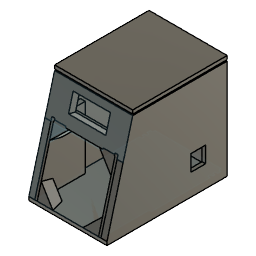
3rd_Seisaku_Alarm (Autodesk Fusion 360 design; units mm, degrees)
Autodesk Fusion 360 part; units mm, degrees
sketch "スケッチ1" plane through (0, 0, 0) normal (0, 0, 1) x (1, 0, 0)
  line L0 (0, 0) -> (3, 0)
  line L1 (3, 0) -> (3, 100)
  line L2 (3, 100) -> (0, 100)
  line L3 (0, 100) -> (0, 0)
  line L4 (3, 100) -> (62, 100)
  line L5 (62, 100) -> (62, 97)
  line L6 (62, 97) -> (3, 97)
  line L7 (3, 97) -> (3, 100)
  line L8 (65.000001, 100.000001) -> (62.000001, 100.000001)
  line L9 (62.000001, 100.000001) -> (62.000001, 0.000001)
  line L10 (62.000001, 0.000001) -> (65.000001, 0.000001)
  line L11 (65.000001, 0.000001) -> (65.000001, 100.000001)
  dimension "d1" = 100
  dimension "d2" = 59
  dimension "d3" = 3
  dimension "d4" = 3
  dimension "d5" = 100
  constraint horizontal L0
  constraint vertical L1
  constraint horizontal L2
  constraint vertical L3
  constraint coincident L0.start L3.end
  constraint horizontal L4
  constraint vertical L5
  constraint horizontal L6
  constraint vertical L7
  constraint horizontal L8
  constraint vertical L9
  constraint horizontal L10
  constraint vertical L11
  measures "d1" distance of L0.start L2.end
  measures "d2" distance of L1.end L4.end
  measures "d3" distance of L1.end L6.end
extrude "押し出し1" add sketch "スケッチ1" along normal blind 80 makes body 1
sketch "スケッチ2" plane through (65.000001, 0, 0) normal (1, 0, 0) x (0, 1, 0)
  line L0 (0.000001, 0) -> (100.000001, 0)
  line L1 (100.000001, 0) -> (100.000001, 80)
  line L2 (100.000001, 80) -> (0.000001, 80)
  line L3 (0.000001, 80) -> (0.000001, 0)
  line L4 (0.000001, 0) -> (22.116636, 82.540402)
  line L5 (0.000001, 0) -> (85.452114, 0) construction
  line L6 (22.116636, 82.540402) -> (0, 82.540402)
  line L7 (0, 82.540402) -> (0.000001, 0)
  dimension "d8" = 75
  constraint horizontal L5
  constraint perpendicular L3 L6
  measures "d8" angle of L4 L5
extrude "押し出し2" cut sketch "スケッチ2" against normal blind 115 contours L2 L3 L4 L7 picked at (7.145313, 53.333333) bodies 1
sketch "スケッチ3" plane through (0, 0, 0) normal (0, 0, 1) x (1, 0, 0)
  line L0 (65, 100) -> (0, 100)
  line L1 (0, 100) -> (0, 0)
  line L2 (0, 0) -> (65, 0)
  line L3 (65, 0) -> (65, 100)
  constraint horizontal L0
  constraint vertical L1
  constraint horizontal L2
  constraint vertical L3
  constraint coincident L1.end L2.start
extrude "押し出し3" add sketch "スケッチ3" against normal blind 3 bodies 1
sketch "スケッチ4" plane through (0, 0, 0) normal (0, 1, 0) x (1, 0, 0)
  line L0 (0, 0) -> (5, 0)
  line L1 (5, 0) -> (5, -50)
  line L2 (5, -50) -> (0, -50)
  line L3 (0, -50) -> (0, 0)
  line L4 (65.000001, 0) -> (60.000001, 0)
  line L5 (60.000001, 0) -> (60.000001, -50)
  line L6 (60.000001, -50) -> (65.000001, -50)
  line L7 (65.000001, -50) -> (65.000001, 0)
  dimension "d13" = 5
  dimension "d14" = 50
  dimension "d15" = 5
  dimension "d16" = 50
  constraint horizontal L0
  constraint vertical L1
  constraint horizontal L2
  constraint vertical L3
  constraint coincident L0.start L3.end
  constraint horizontal L4
  constraint vertical L5
  constraint horizontal L6
  constraint vertical L7
  measures "d13" distance of L0.start L0.end
  measures "d14" distance of L0.start L2.end
extrude "押し出し4" add sketch "スケッチ4" along normal blind 40 bodies 1
sketch "スケッチ5" plane through (65.000001, 0, 0) normal (1, 0, 0) x (0, 1, 0)
  line L0 (0, 50) -> (0, -3)
  line L1 (0, -3) -> (100, -3)
  line L2 (100, -3) -> (100.000001, 80)
  line L3 (100.000001, 80) -> (21.435937, 80)
  line L4 (21.435937, 80) -> (13.397461, 50)
  line L5 (13.397461, 50) -> (0, 50)
  line L6 (0, 0) -> (14.246435, 53.168413)
  line L7 (14.246435, 53.168413) -> (0, 53.168413)
  line L8 (0, 53.168413) -> (0, 0)
  constraint coincident L6.start L8.end
  constraint parallel L5 L7
  constraint perpendicular L7 L8
extrude "押し出し5" cut sketch "スケッチ5" against normal blind 77 contours L0 L5 L6 L8 picked at (4.46582, 33.333333) bodies 1
sketch "スケッチ6" plane through (0, 0, 0) normal (0, -0.965926, 0.258819) x (1, 0, 0)
  line L0 (5, 0) -> (5, 51.763809)
  line L1 (5, 51.763809) -> (3, 51.763809)
  line L2 (3, 51.763809) -> (0, 51.763809)
  line L3 (0, 51.763809) -> (0, 0)
  line L4 (0, 0) -> (5, 0)
  line L5 (5, 51.763809) -> (17, 51.763809)
  line L6 (5, 51.763809) -> (5, 39.763809)
  line L7 (17, 51.763809) -> (5, 39.763809)
  line L8 (59.943204, 51.763809) -> (47.943204, 51.763809)
  line L9 (59.943204, 51.763809) -> (59.943204, 39.763809)
  line L10 (59.943204, 39.763809) -> (47.943204, 51.763809)
  line L11 (5, 0) -> (5, 12)
  line L12 (5, 0) -> (17, 0)
  line L13 (5, 12) -> (17, 0)
  line L14 (60.000001, 0) -> (48.000001, 0)
  line L15 (60.000001, 0) -> (60.000001, 12)
  line L16 (60.000001, 12) -> (48.000001, 0)
  dimension "d21" = 12
  dimension "d22" = 12
  dimension "d23" = 12
  dimension "d24" = 12
  dimension "d25" = 12
  dimension "d26" = 12
  dimension "d27" = 12
  dimension "d28" = 12
  constraint perpendicular L0 L5
  constraint perpendicular L6 L8
  constraint perpendicular L8 L9
  constraint coincident L0.start L4.end
  constraint perpendicular L4 L11
  constraint perpendicular L11 L12
  constraint perpendicular L11 L14
  constraint perpendicular L14 L15
  measures "d25" distance of L0.start L11.end
  measures "d26" distance of L0.start L12.end
extrude "押し出し6" add sketch "スケッチ6" against normal blind 5 separate body contours L0 L11 L12 L13 | L0 L5 L6 L7 | L8 L9 L10 | L14 L15 L16 picked at (9, 4) picked at (9, 47.763809) picked at (55.943204, 47.763809) picked at (56.000001, 4) makes body 2 at (13, 2.645153, 3.432338) makes body 3 at (56.000001, 3.680429, 7.296042) makes body 4 at (9, 14.546661, 41.409863) makes body 5 at (55.943204, 12.936785, 41.841228)
sketch "スケッチ7" plane through (5, 0, 0) normal (1, 0, 0) x (0, 1, 0)
  line L0 (13.397461, 50) -> (0, 0)
  line L1 (0, 0) -> (40, 0)
  line L2 (40, 0) -> (40, 50)
  line L3 (40, 50) -> (13.397461, 50)
sketch "スケッチ8" plane through (5, 0, 0) normal (1, 0, 0) x (0, 1, 0)
extrude "押し出し7" add 2 faces at (9, 15.007337, 49.568635) (55.943204, 15.007337, 49.568635) along direction (0, 0.25881907, 0.96592582) blind 2 on bodies 4 5 bodies 1 2 3 5 4
sketch "スケッチ9" plane through (0, 0, 0) normal (0, -0.965926, 0.258819) x (1, 0, 0)
  line L0 (5, 51.763809) -> (3, 51.763809)
  line L1 (3, 51.763809) -> (0, 51.763809)
  line L2 (0, 51.763809) -> (0, 0)
  line L3 (0, 0) -> (5, 0)
  line L4 (5, 0) -> (5, 39.763809)
  line L5 (5, 39.763809) -> (17, 51.763809)
  line L6 (17, 51.763809) -> (17, 53.763809)
  line L7 (17, 53.763809) -> (5, 53.763809)
  line L8 (5, 53.763809) -> (5, 51.763809)
  line L9 (3, 51.763809) -> (62.000001, 51.763809)
  line L10 (62.000001, 51.763809) -> (62.000001, 55.000001)
  line L11 (62.000001, 55.000001) -> (3, 55.000001)
  line L12 (3, 55.000001) -> (3, 51.763809)
  constraint horizontal L9
  constraint vertical L10
  constraint horizontal L11
  constraint vertical L12
sketch "スケッチ10" plane through (3, 0, 0) normal (1, 0, 0) x (0, 1, 0)
  line L0 (13.397461, 50) -> (40, 50)
  line L1 (40, 50) -> (40, 0)
  line L2 (40, 0) -> (97, 0)
  line L3 (97, 0) -> (97, 80)
  line L4 (97, 80) -> (21.435937, 80)
  line L5 (21.435937, 80) -> (13.397461, 50)
  line L6 (40, 50) -> (13, 50)
  line L7 (13, 50) -> (13, 53.000001)
  line L8 (13, 53.000001) -> (40, 53.000001)
  line L9 (40, 53.000001) -> (40, 50)
  constraint horizontal L6
  constraint vertical L7
  constraint horizontal L8
  constraint vertical L9
  constraint coincident L0.end L1.start
extrude "押し出し8" add sketch "スケッチ10" along normal blind 59 contours L0 L5 L6 L8 L9 picked at (22.532923, 51) bodies 1 5
sketch "スケッチ11" plane through (0, 0, 53.000001) normal (0, 0, 1) x (-1, 0, 0)
  line L0 (-3, -40) -> (-3, -14.201309)
  line L1 (-3, -14.201309) -> (-62, -14.201309)
  line L2 (-62, -14.201309) -> (-62, -40)
  line L3 (-62, -40) -> (-3, -40)
  line L4 (-62, -40) -> (-3, -40)
  line L5 (-3, -40) -> (-3, -30)
  line L6 (-3, -30) -> (-62, -30)
  line L7 (-62, -30) -> (-62, -40)
  constraint horizontal L4
  constraint vertical L5
  constraint horizontal L6
  constraint vertical L7
  constraint coincident L0 L5.end
  constraint coincident L2.end L3.start
extrude "押し出し9" cut sketch "スケッチ11" against normal blind 3 contours L0 L2 L3 L4 L5 L6 L7 picked at (-42.333333, -36.666667) bodies 1
sketch "スケッチ12" plane through (0, 0, 50.000001) normal (0, 0, 1) x (-1, 0, 0)
  line L0 (-5, -30) -> (-5, -40)
  line L1 (-5, -40) -> (-3, -40)
  line L2 (-3, -40) -> (-3, -30)
  line L3 (-3, -30) -> (-5, -30)
  line L4 (-3, -30) -> (-5, -30)
  line L5 (-5, -30) -> (-5, -40)
  line L6 (-5, -40) -> (-3, -40)
  line L7 (-3, -40) -> (-3, -30)
  line L8 (-60.000001, -40.000001) -> (-62.000001, -40.000001)
  line L9 (-62.000001, -40.000001) -> (-62.000001, -30)
  line L10 (-62.000001, -30) -> (-60.000001, -30)
  line L11 (-60.000001, -30) -> (-60.000001, -40.000001)
  constraint horizontal L4
  constraint vertical L5
  constraint horizontal L6
  constraint vertical L7
  constraint coincident L0.end L1.start
  constraint coincident L2.end L3.start
  constraint horizontal L8
  constraint vertical L9
  constraint horizontal L10
  constraint vertical L11
extrude "押し出し10" add sketch "スケッチ12" along normal blind 3 bodies 1
extrude "押し出し11" cut 1 faces at (42.333333, 97, 26.666667) along direction (0, 1, 0) blind 49 on bodies 1 bodies 1
sketch "スケッチ13" plane through (0, 0.000001, 0) normal (0, -0.965926, 0.258819) x (1, 0, 0)
  line L0 (0, 51.763809) -> (5, 51.763809)
  line L1 (5, 51.763809) -> (5, 53.763809)
  line L2 (5, 53.763809) -> (17, 53.763809)
  line L3 (17, 53.763809) -> (17, 51.763809)
  line L4 (17, 51.763809) -> (47.943204, 51.763809)
  line L5 (47.943204, 51.763809) -> (47.943204, 53.763809)
  line L6 (47.943204, 53.763809) -> (59.943204, 53.763809)
  line L7 (59.943204, 53.763809) -> (59.943204, 51.763809)
  line L8 (59.943204, 51.763809) -> (60.000001, 51.763809)
  line L9 (60.000001, 51.763809) -> (65.000001, 51.763809)
  line L10 (65.000001, 51.763809) -> (65.000001, 82.822095)
  line L11 (65.000001, 82.822095) -> (62.000001, 82.822095)
  line L12 (62.000001, 82.822095) -> (62, 54.869639)
  line L13 (62, 54.869639) -> (3, 54.869639)
  line L14 (3, 54.869639) -> (3, 82.822095)
  line L15 (3, 82.822095) -> (0, 82.822095)
  line L16 (0, 82.822095) -> (0, 51.763809)
sketch "スケッチ14" plane through (0, 0.000001, 0) normal (0, -0.965926, 0.258819) x (1, 0, 0)
sketch "スケッチ15" plane through (0, 0.000001, 0) normal (0, -0.965926, 0.258819) x (1, 0, 0)
sketch "スケッチ16" plane through (0, 0.000001, 0) normal (0, -0.965926, 0.258819) x (1, 0, 0)
sketch "スケッチ17" plane through (0, 0.000001, 0) normal (0, -0.965926, 0.258819) x (1, 0, 0)
  line L0 (17, 62.000001) -> (48, 62.000001)
  line L1 (48, 62.000001) -> (48, 77.000001)
  line L2 (48, 77.000001) -> (17, 77.000001)
  line L3 (17, 77.000001) -> (17, 62.000001)
  line L4 (3, 55.000001) -> (62.000001, 55.000001)
  line L5 (62.000001, 55.000001) -> (62.000001, 83.000001)
  line L6 (62.000001, 83.000001) -> (3, 83.000001)
  line L7 (3, 83.000001) -> (3, 55.000001)
  dimension "d43" = 31
  dimension "d44" = 15
  constraint horizontal L0
  constraint vertical L1
  constraint horizontal L2
  constraint vertical L3
  constraint horizontal L4
  constraint vertical L5
  constraint horizontal L6
  constraint vertical L7
extrude "押し出し12" add sketch "スケッチ17" against normal blind 6 bodies 1
sketch "スケッチ18" plane through (0, 0, 0) normal (0, 0, 1) x (-1, 0, 0)
  line L0 (-60.000001, -40) -> (-62.000001, -40)
  line L1 (-62.000001, -40) -> (-62.000001, -100.000001)
  line L2 (-62.000001, -100.000001) -> (-3, -100.000001)
  line L3 (-3, -100.000001) -> (-3, -40)
  line L4 (-3, -40) -> (-5, -40)
  line L5 (-5, -40) -> (-5, 0)
  line L6 (-5, 0) -> (-60.000001, 0)
  line L7 (-60.000001, 0) -> (-60.000001, -40)
  line L8 (-5, -98.000001) -> (-3, -98.000001)
  line L9 (-3, -98.000001) -> (-3, -100.000001)
  line L10 (-3, -100.000001) -> (-5, -100.000001)
  line L11 (-5, -100.000001) -> (-5, -98.000001)
  line L12 (-5, -95.000001) -> (-3, -95.000001)
  line L13 (-3, -95.000001) -> (-3, -93.000001)
  line L14 (-3, -93.000001) -> (-5, -93.000001)
  line L15 (-5, -93.000001) -> (-5, -95.000001)
  line L16 (-62.000001, -100.000001) -> (-60.000001, -100.000001)
  line L17 (-60.000001, -100.000001) -> (-60.000001, -98.000001)
  line L18 (-60.000001, -98.000001) -> (-62.000001, -98.000001)
  line L19 (-62.000001, -98.000001) -> (-62.000001, -100.000001)
  line L20 (-62.000001, -95.000001) -> (-60.000001, -95.000001)
  line L21 (-60.000001, -95.000001) -> (-60.000001, -93.000001)
  line L22 (-60.000001, -93.000001) -> (-62.000001, -93.000001)
  line L23 (-62.000001, -93.000001) -> (-62.000001, -95.000001)
  line L24 (-3, -91.000001) -> (-5, -91.000001)
  line L25 (-5, -91.000001) -> (-5, -89.000001)
  line L26 (-5, -89.000001) -> (-3, -89.000001)
  line L27 (-3, -89.000001) -> (-3, -91.000001)
  line L28 (-62.000001, -91.000001) -> (-60.000001, -91.000001)
  line L29 (-60.000001, -91.000001) -> (-60.000001, -89.000001)
  line L30 (-60.000001, -89.000001) -> (-62.000001, -89.000001)
  line L31 (-62.000001, -89.000001) -> (-62.000001, -91.000001)
  constraint horizontal L8
  constraint vertical L9
  constraint horizontal L10
  constraint vertical L11
  constraint horizontal L12
  constraint vertical L13
  constraint horizontal L14
  constraint vertical L15
  constraint horizontal L16
  constraint vertical L17
  constraint horizontal L18
  constraint vertical L19
  constraint horizontal L20
  constraint vertical L21
  constraint horizontal L22
  constraint vertical L23
  constraint horizontal L24
  constraint vertical L25
  constraint horizontal L26
  constraint vertical L27
  constraint horizontal L28
  constraint vertical L29
  constraint horizontal L30
  constraint vertical L31
extrude "押し出し13" add sketch "スケッチ18" along normal blind 80 contours L1 L28 L29 L30 L31 | L1 L20 L21 L22 L23 | L3 L24 L25 L26 L27 | L1 L2 L16 L17 L18 L19 | L3 L12 L13 L14 L15 | L2 L3 L8 L9 L10 L11 picked at (-61.333334, -89.666668) picked at (-61.333334, -93.666668) picked at (-4.333333, -89.666668) picked at (-61.333334, -98.666668) picked at (-4.333333, -93.666668) picked at (-4.333333, -98.666668) bodies 1
extrude "押し出し14" add 1 faces at (22.666667, 14.391696, 53.083948) along direction (0, -0.25881905, -0.96592583) blind 0.5 on bodies 1 bodies 1
sketch "スケッチ19" plane through (62.000001, 0, 0) normal (-1, 0, 0) x (0, -1, 0)
  line L0 (-89.000001, 80) -> (-89.000001, 0)
  line L1 (-89.000001, 0) -> (-40, 0)
  line L2 (-40, 0) -> (-40.000001, 53.000001)
  line L3 (-40.000001, 53.000001) -> (-20.412966, 53.000001)
  line L4 (-20.412966, 53.000001) -> (-27.277537, 78.61893)
  line L5 (-27.277537, 78.61893) -> (-22.123315, 80)
  line L6 (-22.123315, 80) -> (-89.000001, 80)
  line L7 (-27.277537, 78.61893) -> (-27.277537, 80)
  line L8 (-27.277537, 78.61893) -> (-22.123315, 80)
  line L9 (-27.277537, 80) -> (-22.123315, 80)
  constraint perpendicular L6 L7
extrude "押し出し15" add sketch "スケッチ19" along normal blind 59 contours L5 L6 L7 L8 L9 picked at (-25.559463, 79.539643) bodies 1
sketch "スケッチ20" plane through (0, 0, 0) normal (-1, 0, 0) x (0, -1, 0)
  line L0 (0, 0) -> (-13.397461, 50)
  line L1 (-13.397461, 50) -> (-21.435937, 80)
  line L2 (-21.435937, 80) -> (-100, 80)
  line L3 (-100, 80) -> (-100, -3)
  line L4 (-100, -3) -> (0, -3)
  line L5 (0, -3) -> (0, 0)
  line L6 (-20, 80.000001) -> (-23.698632, 80.000001)
  line L7 (-23.698632, 80.000001) -> (-23.698632, 82.899312)
  line L8 (-23.698632, 82.899312) -> (-20, 82.899312)
  line L9 (-20, 82.899312) -> (-20, 80.000001)
  constraint horizontal L6
  constraint vertical L7
  constraint horizontal L8
  constraint vertical L9
extrude "押し出し16" cut sketch "スケッチ20" against normal blind 378 contours L2 L6 L7 L8 L9 picked at (-21.711523, 81.932875) bodies 1
sketch "スケッチ21" plane through (0, 5.795556, -1.552915) normal (0, 0.965926, -0.258819) x (-1, 0, 0)
  line L0 (-62.000001, 56.477334) -> (-3, 56.477334)
  line L1 (-3, 56.477334) -> (-3, 83.000001)
  line L2 (-3, 83.000001) -> (-62.000001, 83.000001)
  line L3 (-62.000001, 83.000001) -> (-62.000001, 56.477334)
  line L4 (-17, 77.000001) -> (-17, 62.000001)
  line L5 (-17, 62.000001) -> (-48, 62.000001)
  line L6 (-48, 62.000001) -> (-48, 77.000001)
  line L7 (-48, 77.000001) -> (-17, 77.000001)
  line L8 (-48, 77.000001) -> (-41.000001, 77.000001)
  line L9 (-41.000001, 77.000001) -> (-41.000001, 79.000001)
  circle A0 centre (-41.000001, 79.000001) radius 1
  dimension "d56" = 2
  constraint perpendicular L8 L9
  measures "d56" diameter of A0
extrude "押し出し17" cut sketch "スケッチ21" against normal blind 6 contours A0 picked at (-40.876486, 78.703421) bodies 1
sketch "スケッチ22" plane through (0, 0, 0) normal (0, 1, 0) x (1, 0, 0)
sketch "スケッチ23" plane through (0, 0.000001, 0) normal (0, -0.965926, 0.258819) x (1, 0, 0)
  circle A0 centre (41.000001, 79.000001) radius 1
  line L0 (65.000001, 82.822095) -> (0, 82.822095)
  line L1 (0, 82.822095) -> (0, 51.763809)
  line L2 (0, 51.763809) -> (5, 51.763809)
  line L3 (5, 51.763809) -> (5, 53.763809)
  line L4 (5, 53.763809) -> (17, 53.763809)
  line L5 (17, 53.763809) -> (17, 51.763809)
  line L6 (17, 51.763809) -> (47.943204, 51.763809)
  line L7 (47.943204, 51.763809) -> (47.943204, 53.763809)
  line L8 (47.943204, 53.763809) -> (59.943204, 53.763809)
  line L9 (59.943204, 53.763809) -> (59.943204, 51.763809)
  line L10 (59.943204, 51.763809) -> (60.000001, 51.763809)
  line L11 (60.000001, 51.763809) -> (65.000001, 51.763809)
  line L12 (65.000001, 51.763809) -> (65.000001, 82.822095)
  line L13 (17, 62.000001) -> (17, 77.000001)
  line L14 (17, 77.000001) -> (48, 77.000001)
  line L15 (48, 77.000001) -> (48, 62.000001)
  line L16 (48, 62.000001) -> (17, 62.000001)
  circle A1 centre (41.000001, 79.000001) radius 0.999997
  constraint concentric A0 A1
extrude "押し出し18" add sketch "スケッチ23" against normal blind 6 contours A0 A1 picked at (41.08526, 79.47291) bodies 1
sketch "スケッチ24" plane through (0, 0, 0) normal (0, -0.965926, 0.258819) x (1, 0, 0)
  line L0 (5, 51.763809) -> (0, 51.763809)
  line L1 (0, 51.763809) -> (0, 0)
  line L2 (0, 0) -> (5, 0)
  line L3 (5, 0) -> (5, 39.763809)
  line L4 (5, 39.763809) -> (17, 51.763809)
  line L5 (17, 51.763809) -> (17, 53.763809)
  line L6 (17, 53.763809) -> (5, 53.763809)
  line L7 (5, 53.763809) -> (5, 51.763809)
sketch "スケッチ25" plane through (0, 0, 0) normal (0, 0, 1) x (-1, 0, 0)
  line L0 (-5, -98.000001) -> (-3, -98.000001)
  line L1 (-3, -98.000001) -> (-3, -95.000001)
  line L2 (-3, -95.000001) -> (-5, -95.000001)
  line L3 (-5, -95.000001) -> (-5, -93.000001)
  line L4 (-5, -93.000001) -> (-3, -93.000001)
  line L5 (-3, -93.000001) -> (-3, -91.000001)
  line L6 (-3, -91.000001) -> (-5, -91.000001)
  line L7 (-5, -91.000001) -> (-5, -89.000001)
  line L8 (-5, -89.000001) -> (-3, -89.000001)
  line L9 (-3, -89.000001) -> (-3, -40)
  line L10 (-3, -40) -> (-5, -40)
  line L11 (-5, -40) -> (-5, 0)
  line L12 (-5, 0) -> (-60.000001, 0)
  line L13 (-60.000001, 0) -> (-60.000001, -40)
  line L14 (-60.000001, -40) -> (-62.000001, -40)
  line L15 (-62.000001, -40) -> (-62.000001, -89.000001)
  line L16 (-62.000001, -89.000001) -> (-60.000001, -89.000001)
  line L17 (-60.000001, -89.000001) -> (-60.000001, -91.000001)
  line L18 (-60.000001, -91.000001) -> (-62.000001, -91.000001)
  line L19 (-62.000001, -91.000001) -> (-62.000001, -93.000001)
  line L20 (-62.000001, -93.000001) -> (-60.000001, -93.000001)
  line L21 (-60.000001, -93.000001) -> (-60.000001, -95.000001)
  line L22 (-60.000001, -95.000001) -> (-62.000001, -95.000001)
  line L23 (-62.000001, -95.000001) -> (-62.000001, -98.000001)
  line L24 (-62.000001, -98.000001) -> (-60.000001, -98.000001)
  line L25 (-60.000001, -98.000001) -> (-60.000001, -100.000001)
  line L26 (-60.000001, -100.000001) -> (-5, -100.000001)
  line L27 (-5, -100.000001) -> (-5, -98.000001)
sketch "スケッチ26" plane through (0, 0, 0) normal (0, 1, 0) x (1, 0, 0)
  line L0 (5, 0) -> (60.000001, 0)
  line L1 (60.000001, 0) -> (60.000001, -50.000001)
  line L2 (60.000001, -50.000001) -> (5, -50.000001)
  line L3 (5, -50.000001) -> (5, 0)
  constraint horizontal L0
  constraint vertical L1
  constraint horizontal L2
  constraint vertical L3
extrude "押し出し19" cut sketch "スケッチ26" along normal blind 39 bodies 1 2 3
sketch "スケッチ27" plane through (0, 0, 0) normal (0, 0, 1) x (-1, 0, 0)
  line L0 (-5, 0) -> (-7.5, 0)
  line L1 (-7.5, 0) -> (-7.5, -40.000001)
  line L2 (-7.5, -40.000001) -> (-5, -40.000001)
  line L3 (-5, -40.000001) -> (-5, 0)
  line L4 (-60.000001, -40.000001) -> (-57.500001, -40.000001)
  line L5 (-57.500001, -40.000001) -> (-57.500001, -0.000001)
  line L6 (-57.500001, -0.000001) -> (-60.000001, -0.000001)
  line L7 (-60.000001, -0.000001) -> (-60.000001, -40.000001)
  dimension "d63" = 2.5
  dimension "d64" = 2.5
  dimension "d65" = 40
  constraint horizontal L0
  constraint vertical L1
  constraint horizontal L2
  constraint vertical L3
  constraint horizontal L4
  constraint vertical L5
  constraint horizontal L6
  constraint vertical L7
  measures "d63" distance of L0.start L0.end
extrude "押し出し20" add sketch "スケッチ27" along normal blind 53 bodies 1 2 3
sketch "スケッチ28" plane through (65.000001, 0, 0) normal (1, 0, 0) x (0, 1, 0)
  line L0 (13.397461, 50) -> (0, 0)
  line L1 (0, 0) -> (0, -3)
  line L2 (0, -3) -> (100, -3)
  line L3 (100, -3) -> (100.000001, 80)
  line L4 (100.000001, 80) -> (21.435937, 80)
  line L5 (21.435937, 80) -> (13.397461, 50)
  line L6 (21.435937, 80) -> (0, 0)
  line L7 (0, 80.000001) -> (21.435937, 80)
  line L8 (0, 80.000001) -> (0, 0)
  constraint coincident L0.end L1.start
  constraint parallel L1 L8
extrude "押し出し21" cut sketch "スケッチ28" against normal blind 541 contours L0 L5 L6 L7 L8 picked at (11.611133, 70) bodies 1
extrude "押し出し22" cut 1 faces at (7.5, 19.524614, 16.666667) along direction (-1, 0, 0) blind 0.5 on bodies 1 bodies 1
extrude "押し出し23" cut 1 faces at (57.500001, 19.524614, 16.666667) along direction (1, 0, 0) blind 0.5 on bodies 1 bodies 1
sketch "スケッチ29" plane through (0, 0.000001, 0) normal (0, -0.965926, 0.258819) x (1, 0, 0)
  line L0 (17, 62.000001) -> (17, 77.000001)
  line L1 (17, 77.000001) -> (48, 77.000001)
  line L2 (48, 77.000001) -> (48, 62.000001)
  line L3 (48, 62.000001) -> (17, 62.000001)
  line L4 (57.500001, 53.763809) -> (57.500001, 54.869638)
  line L5 (57.500001, 54.869638) -> (60.000001, 54.869638)
  line L6 (60.000001, 54.869638) -> (60.000001, 51.763809)
  line L7 (60.000001, 51.763809) -> (65.000001, 51.763809)
  line L8 (65.000001, 51.763809) -> (65.000001, 82.822095)
  line L9 (65.000001, 82.822095) -> (0, 82.822095)
  line L10 (0, 82.822095) -> (0, 51.763809)
  line L11 (0, 51.763809) -> (5, 51.763809)
  line L12 (5, 51.763809) -> (5, 53.763809)
  line L13 (5, 53.763809) -> (5, 54.869638)
  line L14 (5, 54.869638) -> (7.5, 54.869638)
  line L15 (7.5, 54.869638) -> (7.5, 53.763809)
  line L16 (7.5, 53.763809) -> (17, 53.763809)
  line L17 (17, 53.763809) -> (17, 51.763809)
  line L18 (17, 51.763809) -> (47.943204, 51.763809)
  line L19 (47.943204, 51.763809) -> (47.943204, 53.763809)
  line L20 (47.943204, 53.763809) -> (57.500001, 53.763809)
  line L21 (7, 0) -> (20, 0)
  line L22 (7, 0) -> (7, 0.338303)
  line L23 (7, 0) -> (7, 13)
  line L24 (7, 13) -> (20, 0)
  line L25 (58.000001, 0) -> (45.000001, 0)
  line L26 (58.000001, 0) -> (58.000001, 13)
  line L27 (58.000001, 13) -> (45.000001, 0)
  line L28 (7, 51.500001) -> (7, 38.500001)
  line L29 (7, 51.500001) -> (20, 51.500001)
  line L30 (20, 51.500001) -> (7, 38.500001)
  line L31 (58.000001, 51.500001) -> (45.000001, 51.500001)
  line L32 (58.000001, 51.500001) -> (58.000001, 38.500001)
  line L33 (45.000001, 51.500001) -> (58.000001, 38.500001)
  dimension "d74" = 13
  dimension "d75" = 13
  dimension "d76" = 13
  dimension "d77" = 13
  dimension "d78" = 13
  dimension "d79" = 13
  dimension "d80" = 13
  dimension "d81" = 13
  constraint horizontal L21
  constraint perpendicular L21 L22
  constraint perpendicular L21 L23
  constraint perpendicular L23 L25
  constraint perpendicular L25 L26
  constraint parallel L10 L28
  constraint perpendicular L28 L29
  constraint perpendicular L19 L31
  constraint perpendicular L31 L32
  measures "d74" distance of L21.start L21.end
  measures "d75" distance of L21.start L23.end
extrude "押し出し24" add sketch "スケッチ29" against normal blind 10 contours L21 L22 L23 L24 | L25 L26 L27 | L28 L29 L30 | L31 L32 L33 picked at (11.333333, 4.446101) picked at (53.666668, 4.333333) picked at (11.333333, 47.166667) picked at (53.666668, 47.166667) bodies 1
sketch "スケッチ30" plane through (58.000001, 0, 0) normal (-1, 0, 0) x (0, -1, 0)
  line L0 (-22.988441, 47.15699) -> (-13.329182, 49.74518)
  line L1 (-13.329182, 49.74518) -> (-13.397461, 50.000001)
  line L2 (-13.397461, 50.000001) -> (-30, 50)
  line L3 (-30, 50) -> (-30, 53)
  line L4 (-30, 53) -> (-40.000001, 53)
  line L5 (-40.000001, 53) -> (-40.000001, 0)
  line L6 (-40.000001, 0) -> (-10.352763, 0)
  line L7 (-10.352763, 0) -> (-13.023907, 9.968845)
  line L8 (-13.023907, 9.968845) -> (-3.364649, 12.557035)
  line L9 (-3.364649, 12.557035) -> (-9.964535, 37.188145)
  line L10 (-9.964535, 37.188145) -> (-19.623793, 34.599954)
  line L11 (-19.623793, 34.599954) -> (-22.988441, 47.15699)
  line L12 (-22.988441, 47.15699) -> (-22.988441, 50)
  line L13 (-22.988441, 47.15699) -> (-13.329182, 49.74518)
  line L14 (-22.988441, 50) -> (-13.397461, 50.000001)
  constraint perpendicular L2 L12
extrude "押し出し25" add sketch "スケッチ30" along normal blind 51 contours L0 L1 L2 L12 L13 L14 picked at (-19.768688, 48.96739) bodies 1
sketch "スケッチ31" plane through (0, 0, 0) normal (0, 1, 0) x (1, 0, 0)
  line L0 (20, -50.000001) -> (45.000001, -50.000001)
  line L1 (45.000001, -50.000001) -> (45.000001, -47.000001)
  line L2 (45.000001, -47.000001) -> (20, -47.000001)
  line L3 (20, -47.000001) -> (20, -50.000001)
  constraint horizontal L0
  constraint vertical L1
  constraint horizontal L2
  constraint vertical L3
extrude "押し出し26" cut sketch "スケッチ31" along normal blind 145 bodies 1
sketch "スケッチ32" plane through (0, 0.000001, 0) normal (0, -0.965926, 0.258819) x (1, 0, 0)
  line L0 (17, 62.000001) -> (17, 77.000001)
  line L1 (17, 77.000001) -> (48, 77.000001)
  line L2 (48, 77.000001) -> (48, 62.000001)
  line L3 (48, 62.000001) -> (17, 62.000001)
  line L4 (57.500001, 53.763809) -> (57.500001, 54.869638)
  line L5 (57.500001, 54.869638) -> (60.000001, 54.869638)
  line L6 (60.000001, 54.869638) -> (60.000001, 51.763809)
  line L7 (60.000001, 51.763809) -> (65.000001, 51.763809)
  line L8 (65.000001, 51.763809) -> (65.000001, 82.822095)
  line L9 (65.000001, 82.822095) -> (0, 82.822095)
  line L10 (0, 82.822095) -> (0, 51.763809)
  line L11 (0, 51.763809) -> (5, 51.763809)
  line L12 (5, 51.763809) -> (5, 53.763809)
  line L13 (5, 53.763809) -> (5, 54.869638)
  line L14 (5, 54.869638) -> (7.5, 54.869638)
  line L15 (7.5, 54.869638) -> (7.5, 53.763809)
  line L16 (7.5, 53.763809) -> (17, 53.763809)
  line L17 (17, 53.763809) -> (17, 51.763809)
  line L18 (17, 51.763809) -> (20, 51.76381)
  line L19 (20, 51.76381) -> (45.000001, 51.76381)
  line L20 (45.000001, 51.76381) -> (47.943204, 51.763809)
  line L21 (47.943204, 51.763809) -> (47.943204, 53.763809)
  line L22 (47.943204, 53.763809) -> (57.500001, 53.763809)
sketch "スケッチ33" plane through (0, 0, 0) normal (0, 1, 0) x (1, 0, 0)
sketch "スケッチ34" plane through (0, 40, 0) normal (0, 1, 0) x (-1, 0, 0)
  line L0 (-7, 53) -> (-7, 0)
  line L1 (-7, 0) -> (-3, 0)
  line L2 (-3, 0) -> (-3, 53.000001)
  line L3 (-3, 53.000001) -> (-7, 53)
  line L4 (-3, 52.000001) -> (-62.000001, 52.000001)
  line L5 (-62.000001, 52.000001) -> (-62.000001, 53.000001)
  line L6 (-62.000001, 53.000001) -> (-3, 53.000001)
  line L7 (-3, 53.000001) -> (-3, 52.000001)
  constraint horizontal L4
  constraint vertical L5
  constraint horizontal L6
  constraint vertical L7
extrude "押し出し27" cut sketch "スケッチ34" against normal blind 19 contours L0 L2 L3 L4 L6 L7 | L0 L4 L5 L6 picked at (-4.333333, 52.666667) picked at (-43.666667, 52.666667) bodies 1
sketch "スケッチ35" plane through (0, 0, 0) normal (0, 0, 1) x (-1, 0, 0)
  line L0 (-3, -91.000001) -> (-62.000001, -91.000001)
  line L1 (-62.000001, -91.000001) -> (-62.000001, -89.000001)
  line L2 (-62.000001, -89.000001) -> (-3, -89.000001)
  line L3 (-3, -89.000001) -> (-3, -91.000001)
  constraint horizontal L0
  constraint vertical L1
  constraint horizontal L2
  constraint vertical L3
extrude "押し出し28" cut sketch "スケッチ35" along normal blind 120 bodies 1
sketch "スケッチ36" plane through (0, 0, 0) normal (0, 0, 1) x (-1, 0, 0)
  line L0 (-5, -92.000001) -> (-3, -92.000001)
  line L1 (-3, -92.000001) -> (-3, -93.000001)
  line L2 (-3, -93.000001) -> (-5, -93.000001)
  line L3 (-5, -93.000001) -> (-5, -92.000001)
  line L4 (-60.000001, -92.000001) -> (-62.000001, -92.000001)
  line L5 (-62.000001, -92.000001) -> (-62.000001, -93.000001)
  line L6 (-62.000001, -93.000001) -> (-60.000001, -93.000001)
  line L7 (-60.000001, -93.000001) -> (-60.000001, -92.000001)
  line L8 (-5, -90.000001) -> (-3, -90.000001)
  line L9 (-3, -90.000001) -> (-3, -88.000001)
  line L10 (-3, -88.000001) -> (-5, -88.000001)
  line L11 (-5, -88.000001) -> (-5, -90.000001)
  line L12 (-60.000001, -88.000001) -> (-62.000001, -88.000001)
  line L13 (-62.000001, -88.000001) -> (-62.000001, -90.000001)
  line L14 (-62.000001, -90.000001) -> (-60.000001, -90.000001)
  line L15 (-60.000001, -90.000001) -> (-60.000001, -88.000001)
  constraint horizontal L0
  constraint vertical L1
  constraint horizontal L2
  constraint vertical L3
  constraint horizontal L4
  constraint vertical L5
  constraint horizontal L6
  constraint vertical L7
  constraint horizontal L8
  constraint vertical L9
  constraint horizontal L10
  constraint vertical L11
  constraint horizontal L12
  constraint vertical L13
  constraint horizontal L14
  constraint vertical L15
extrude "押し出し29" add sketch "スケッチ36" along normal blind 80 bodies 1
sketch "スケッチ37" plane through (0, 0, 80) normal (0, 0, 1) x (-1, 0, 0)
  line L0 (-3.000001, -27.277537) -> (-3, -88.000001)
  line L1 (-3, -88.000001) -> (-5, -88.000001)
  line L2 (-5, -88.000001) -> (-5, -90.000001)
  line L3 (-5, -90.000001) -> (-3, -90.000001)
  line L4 (-3, -90.000001) -> (-3, -92.000001)
  line L5 (-3, -92.000001) -> (-5, -92.000001)
  line L6 (-5, -92.000001) -> (-5, -95.000001)
  line L7 (-5, -95.000001) -> (-3, -95.000001)
  line L8 (-3, -95.000001) -> (-3, -98.000001)
  line L9 (-3, -98.000001) -> (-5, -98.000001)
  line L10 (-5, -98.000001) -> (-5, -100.000001)
  line L11 (-5, -100.000001) -> (0, -100)
  line L12 (0, -100) -> (0, -21.435937)
  line L13 (0, -21.435937) -> (-65.000001, -21.435937)
  line L14 (-65.000001, -21.435937) -> (-65.000001, -100.000001)
  line L15 (-65.000001, -100.000001) -> (-60.000001, -100.000001)
  line L16 (-60.000001, -100.000001) -> (-60.000001, -98.000001)
  line L17 (-60.000001, -98.000001) -> (-62.000001, -98.000001)
  line L18 (-62.000001, -98.000001) -> (-62.000001, -95.000001)
  line L19 (-62.000001, -95.000001) -> (-60.000001, -95.000001)
  line L20 (-60.000001, -95.000001) -> (-60.000001, -92.000001)
  line L21 (-60.000001, -92.000001) -> (-62.000001, -92.000001)
  line L22 (-62.000001, -92.000001) -> (-62.000001, -90.000001)
  line L23 (-62.000001, -90.000001) -> (-60.000001, -90.000001)
  line L24 (-60.000001, -90.000001) -> (-60.000001, -88.000001)
  line L25 (-60.000001, -88.000001) -> (-62.000001, -88.000001)
  line L26 (-62.000001, -88.000001) -> (-62.000001, -27.277537)
  line L27 (-62.000001, -27.277537) -> (-3.000001, -27.277537)
  line L28 (-65.000001, -100.000001) -> (0, -100.000001)
  line L29 (0, -100.000001) -> (0, -21.435937)
  line L30 (0, -21.435937) -> (-65.000001, -21.435937)
  line L31 (-65.000001, -21.435937) -> (-65.000001, -100.000001)
  constraint horizontal L28
  constraint vertical L29
  constraint horizontal L30
  constraint vertical L31
extrude "押し出し1'" add sketch "スケッチ37" along normal blind 3 separate body makes body 6 in component "Component"
sketch "スケッチ38" plane through (0, 0, 80) normal (0, 0, -1) x (1, 0, 0)
  line L0 (65.000001, -100.000001) -> (65.000001, -21.435937)
  line L1 (65.000001, -21.435937) -> (0, -21.435937)
  line L2 (0, -21.435937) -> (0, -100.000001)
  line L3 (0, -100.000001) -> (65.000001, -100.000001)
  line L4 (3, -95.499998) -> (63, -95.499998)
  line L5 (63, -95.499998) -> (63, -97.499998)
  line L6 (63, -97.499998) -> (3, -97.499998)
  line L7 (3, -97.499998) -> (3, -95.499998)
  line L8 (63, -95.499998) -> (62, -95.499998)
  line L9 (62, -95.499998) -> (62, -97.499998)
  line L10 (62, -97.499998) -> (63, -97.499998)
  line L11 (63, -97.499998) -> (63, -95.499998)
  dimension "d98" = 60
  dimension "d99" = 2
  dimension "d100" = 1
  constraint horizontal L4
  constraint vertical L5
  constraint horizontal L6
  constraint vertical L7
  constraint horizontal L8
  constraint vertical L9
  constraint horizontal L10
  constraint vertical L11
extrude "押し出し2'" add sketch "スケッチ38" along normal blind 80 contours L4 L6 L7 L9 picked at (22.666667, -96.833331) bodies 6 in component "Component"
sketch "スケッチ39" plane through (62.000001, 0, 0) normal (-1, 0, 0) x (0, -1, 0)
  line L0 (-88.000001, 80) -> (-88.000001, 0)
  line L1 (-88.000001, 0) -> (-40, 0)
  line L2 (-40, 0) -> (-40, 52.000001)
  line L3 (-40, 52.000001) -> (-21, 52.000001)
  line L4 (-21, 52.000001) -> (-21, 53.000001)
  line L5 (-21, 53.000001) -> (-20.412966, 53.000001)
  line L6 (-20.412966, 53.000001) -> (-27.277537, 78.61893)
  line L7 (-27.277537, 78.61893) -> (-27.277537, 80)
  line L8 (-27.277537, 80) -> (-88.000001, 80)
  line L9 (-88.000001, 0) -> (-82.000001, 0)
  line L10 (-82.000001, 0) -> (-71.000001, 0)
  line L11 (-71.000001, 0) -> (-71.000001, 15)
  line L12 (-71.000001, 15) -> (-82.000001, 15)
  line L13 (-82.000001, 15) -> (-82.000001, 28.4)
  line L14 (-82.000001, 28.4) -> (-71.000001, 28.4)
  line L15 (-71.000001, 28.4) -> (-71.000001, 15)
  dimension "d103" = 11
  dimension "d104" = 15
  dimension "d105" = 11
  dimension "d106" = 13.4
  constraint parallel L1 L10
  constraint perpendicular L10 L11
  constraint horizontal L12
  constraint vertical L13
  constraint horizontal L14
  constraint vertical L15
extrude "押し出し30" cut sketch "スケッチ39" against normal blind 5 contours L12 L13 L14 L15 picked at (-74.666668, 19.466667) bodies 1
sketch "スケッチ40" plane through (3, 0, 0) normal (1, 0, 0) x (0, 1, 0)
  line L0 (88.000001, 0) -> (88.000001, 80)
  line L1 (88.000001, 80) -> (27.277537, 80)
  line L2 (27.277537, 80) -> (27.277537, 78.61893)
  line L3 (27.277537, 78.61893) -> (20.412966, 53.000001)
  line L4 (20.412966, 53.000001) -> (21, 53.000001)
  line L5 (21, 53.000001) -> (21, 52.000001)
  line L6 (21, 52.000001) -> (40, 52.000001)
  line L7 (40, 52.000001) -> (40, 0)
  line L8 (40, 0) -> (88.000001, 0)
  line L9 (88.000001, 0) -> (79.000001, 0)
  line L10 (74.000001, 0) -> (74.000001, 11)
  line L11 (74.000001, 11) -> (79.000001, 11)
  line L12 (79.000001, 11) -> (79.000001, 32.4)
  line L13 (79.000001, 32.4) -> (74.000001, 32.4)
  line L14 (74.000001, 32.4) -> (74.000001, 11)
  line L15 (74.000001, 32.4) -> (74.000001, 34.4)
  dimension "d109" = 9
  dimension "d110" = 11
  dimension "d111" = 5
  dimension "d112" = 21.4
  dimension "d115" = 2
  constraint perpendicular L0 L9
  constraint perpendicular L8 L10
  constraint horizontal L11
  constraint vertical L12
  constraint horizontal L13
  constraint vertical L14
  constraint perpendicular L13 L15
extrude "押し出し32" cut sketch "スケッチ40" against normal blind 75 contours L11 L12 L13 L14 picked at (75.666668, 18.133333) bodies 1
sketch "スケッチ41" plane through (0, 0.000001, 0) normal (0, -0.965926, 0.258819) x (1, 0, 0)
  line L0 (7, 51.500001) -> (7, 38.500001)
  line L1 (7, 38.500001) -> (20, 51.500001)
  line L2 (20, 51.500001) -> (7, 51.500001)
sketch "スケッチ42" plane through (7, 0, 0) normal (1, 0, 0) x (0, 1, 0)
  line L0 (40, 52.000001) -> (30, 52.000001)
  line L1 (30, 52.000001) -> (30, 50)
  line L2 (30, 50) -> (22.988441, 50)
  line L3 (22.988441, 50) -> (22.988441, 47.15699)
  line L4 (22.988441, 47.15699) -> (19.623793, 34.599954)
  line L5 (19.623793, 34.599954) -> (9.964535, 37.188145)
  line L6 (9.964535, 37.188145) -> (3.364649, 12.557035)
  line L7 (3.364649, 12.557035) -> (13.023907, 9.968845)
  line L8 (13.023907, 9.968845) -> (10.352763, 0)
  line L9 (10.352763, 0) -> (40.000001, 0)
  line L10 (40.000001, 0) -> (40, 52.000001)
  line L11 (10, 35.000001) -> (28, 35.000001)
  line L12 (28, 35.000001) -> (28, 50.000001)
  line L13 (28, 50.000001) -> (10, 50.000001)
  line L14 (10, 50.000001) -> (10, 35.000001)
  constraint horizontal L11
  constraint vertical L12
  constraint horizontal L13
  constraint vertical L14
extrude "押し出し33" cut sketch "スケッチ42" along normal blind 24 contours L3 L4 L5 L11 L13 L14 picked at (14.32948, 44.778544) bodies 1
sketch "スケッチ43" plane through (7, 0, 0) normal (1, 0, 0) x (0, 1, 0)
  line L0 (19.730985, 35.000001) -> (19.623793, 34.599954)
  line L1 (19.623793, 34.599954) -> (18.1308, 35.000001)
  line L2 (18.1308, 35.000001) -> (19.730985, 35.000001)
  line L3 (30, 50) -> (13.397461, 50.000001)
  line L4 (13.397461, 50.000001) -> (10, 37.320503)
  line L5 (10, 37.320503) -> (10, 37.178642)
  line L6 (10, 37.178642) -> (9.964535, 37.188145)
  line L7 (9.964535, 37.188145) -> (3.364649, 12.557035)
  line L8 (3.364649, 12.557035) -> (13.023907, 9.968845)
  line L9 (13.023907, 9.968845) -> (10.352763, 0)
  line L10 (10.352763, 0) -> (40.000001, 0)
  line L11 (40.000001, 0) -> (40, 52.000001)
  line L12 (40, 52.000001) -> (30, 52.000001)
  line L13 (30, 52.000001) -> (30, 50)
  line L14 (25, 33) -> (3, 33)
  line L15 (3, 33) -> (3, 50.000001)
  line L16 (3, 50.000001) -> (25, 50.000001)
  line L17 (25, 50.000001) -> (25, 33)
  constraint horizontal L14
  constraint vertical L15
  constraint horizontal L16
  constraint vertical L17
sketch "スケッチ44" plane through (7, 0, 0) normal (1, 0, 0) x (0, 1, 0)
  line L0 (20.5, 35.500001) -> (17.5, 35.500001)
  line L1 (17.5, 35.500001) -> (17.5, 34.000001)
  line L2 (17.5, 34.000001) -> (20.5, 34.000001)
  line L3 (20.5, 34.000001) -> (20.5, 35.500001)
  constraint horizontal L0
  constraint vertical L1
  constraint horizontal L2
  constraint vertical L3
extrude "押し出し34" cut sketch "スケッチ44" along normal blind 0.5 bodies 1
extrude "押し出し35" cut sketch "スケッチ43" along normal blind 51 contours L0 L1 L2 | L3 L4 L5 L6 L7 L14 L16 L17 picked at (19.161859, 34.866652) picked at (19.376149, 45.000001) bodies 1
sketch "スケッチ45" plane through (0, 0, 0) normal (0, 1, 0) x (1, 0, 0)
  line L0 (58.000001, -50.000001) -> (7, -50.000001)
  line L1 (7, -50.000001) -> (7, -51.000001)
  line L2 (7, -51.000001) -> (58.000001, -51.000001)
  line L3 (58.000001, -51.000001) -> (58.000001, -50.000001)
  constraint horizontal L0
  constraint vertical L1
  constraint horizontal L2
  constraint vertical L3
extrude "押し出し36" cut sketch "スケッチ45" along normal blind 104 bodies 1
sketch "スケッチ46" plane through (0, 0, 0) normal (0, -0.965926, 0.258819) x (1, 0, 0)
  line L0 (60.000001, 51.763809) -> (60.000001, 0)
  line L1 (60.000001, 0) -> (65.000001, 0)
  line L2 (65.000001, 0) -> (65.000001, 51.763809)
  line L3 (65.000001, 51.763809) -> (60.000001, 51.763809)
  line L4 (58.000001, 53.000001) -> (58.000001, 40.000001)
  line L5 (58.000001, 53.000001) -> (45.000001, 53.000001)
  line L6 (58.000001, 40.000001) -> (45.000001, 53.000001)
  line L7 (7, 53.000001) -> (7, 40.000001)
  line L8 (7, 53.000001) -> (20, 53.000001)
  line L9 (20, 53.000001) -> (7, 40.000001)
  dimension "d126" = 13
  dimension "d127" = 13
  dimension "d128" = 13
  dimension "d129" = 13
  constraint vertical L4
  constraint perpendicular L4 L5
  constraint perpendicular L5 L7
  constraint perpendicular L7 L8
extrude "押し出し37" add sketch "スケッチ46" against normal blind 10 contours L4 L5 L6 | L7 L8 L9 picked at (53.666668, 48.666667) picked at (11.333333, 48.666667) bodies 1
sketch "スケッチ47" plane through (58.000001, 0, 0) normal (-1, 0, 0) x (0, -1, 0)
  line L0 (-10.352763, 38.637034) -> (-20.012021, 36.048843)
  line L1 (-20.012021, 36.048843) -> (-23.376669, 48.605878)
  line L2 (-23.376669, 48.605878) -> (-14.441684, 51.000001)
  line L3 (-14.441684, 51.000001) -> (-30, 51.000001)
  line L4 (-30, 51.000001) -> (-30, 52.000001)
  line L5 (-30, 52.000001) -> (-40, 52.000001)
  line L6 (-40, 52.000001) -> (-40.000001, 0)
  line L7 (-40.000001, 0) -> (-10.352763, 0)
  line L8 (-10.352763, 0) -> (-13.023907, 9.968845)
  line L9 (-13.023907, 9.968845) -> (-3.364649, 12.557035)
  line L10 (-3.364649, 12.557035) -> (-9.964535, 37.188145)
  line L11 (-9.964535, 37.188145) -> (-10, 37.178642)
  line L12 (-10, 37.178642) -> (-10, 37.320503)
  line L13 (-10, 37.320503) -> (-10.352763, 38.637034)
  line L14 (-10.5, 37.500001) -> (-9.5, 37.500001)
  line L15 (-9.5, 37.500001) -> (-9.5, 37.000001)
  line L16 (-9.5, 37.000001) -> (-10.5, 37.000001)
  line L17 (-10.5, 37.000001) -> (-10.5, 37.500001)
  constraint horizontal L14
  constraint vertical L15
  constraint horizontal L16
  constraint vertical L17
extrude "押し出し38" cut sketch "スケッチ47" along normal blind 51 contours L10 L11 L12 L13 L14 L15 L16 | L10 L11 L12 L13 L14 L16 L17 picked at (-9.654845, 37.229382) picked at (-10.333333, 37.273501) bodies 1
sketch "スケッチ48" plane through (0, 0, 0) normal (0, -0.965926, 0.258819) x (1, 0, 0)
sketch "スケッチ49" plane through (7, 0, 0) normal (1, 0, 0) x (0, 1, 0)
  line L0 (10.352763, 38.637034) -> (3.364649, 12.557035)
  line L1 (3.364649, 12.557035) -> (13.023907, 9.968845)
  line L2 (13.023907, 9.968845) -> (10.352763, 0)
  line L3 (10.352763, 0) -> (40.000001, 0)
  line L4 (40.000001, 0) -> (40, 52.000001)
  line L5 (40, 52.000001) -> (30, 52.000001)
  line L6 (30, 52.000001) -> (30, 51.000001)
  line L7 (30, 51.000001) -> (14.441684, 51.000001)
  line L8 (14.441684, 51.000001) -> (23.376669, 48.605878)
  line L9 (23.376669, 48.605878) -> (20.012021, 36.048843)
  line L10 (20.012021, 36.048843) -> (10.352763, 38.637034)
  line L11 (23.376669, 48.605878) -> (24.018172, 51.000001)
  line L12 (14.441684, 51.000001) -> (23.376669, 48.605878)
  constraint perpendicular L8 L11
extrude "押し出し39" add sketch "スケッチ49" along normal blind 13 contours L7 L8 L11 L12 picked at (20.612175, 50.20196) bodies 1
sketch "スケッチ50" plane through (58.000001, 0, 0) normal (-1, 0, 0) x (0, -1, 0)
  line L0 (-3.364649, 12.557035) -> (-10.352763, 38.637034)
  line L1 (-10.352763, 38.637034) -> (-20.012021, 36.048843)
  line L2 (-20.012021, 36.048843) -> (-23.376669, 48.605878)
  line L3 (-23.376669, 48.605878) -> (-14.441684, 51.000001)
  line L4 (-14.441684, 51.000001) -> (-30, 51.000001)
  line L5 (-30, 51.000001) -> (-30, 52.000001)
  line L6 (-30, 52.000001) -> (-40, 52.000001)
  line L7 (-40, 52.000001) -> (-40.000001, 0)
  line L8 (-40.000001, 0) -> (-10.352763, 0)
  line L9 (-10.352763, 0) -> (-13.023907, 9.968845)
  line L10 (-13.023907, 9.968845) -> (-3.364649, 12.557035)
  line L11 (-23.376669, 48.605878) -> (-24.018172, 51.000001)
  line L12 (-14.441684, 51.000001) -> (-23.376669, 48.605878)
  constraint perpendicular L3 L11
extrude "押し出し40" add sketch "スケッチ50" along normal blind 13 contours L3 L4 L11 L12 picked at (-20.612175, 50.20196) bodies 1
sketch "スケッチ51" plane through (62.000001, 0, 0) normal (-1, 0, 0) x (0, -1, 0)
  line L0 (-82.000001, 15) -> (-82.000001, 28.4)
  line L1 (-82.000001, 28.4) -> (-71.000001, 28.4)
  line L2 (-71.000001, 28.4) -> (-71.000001, 15)
  line L3 (-71.000001, 15) -> (-82.000001, 15)
  line L4 (-88.000001, 80) -> (-88.000001, 0)
  line L5 (-88.000001, 0) -> (-40, 0)
  line L6 (-40, 0) -> (-40, 52.000001)
  line L7 (-40, 52.000001) -> (-21, 52.000001)
  line L8 (-21, 52.000001) -> (-21, 53.000001)
  line L9 (-21, 53.000001) -> (-20.412966, 53.000001)
  line L10 (-20.412966, 53.000001) -> (-27.277537, 78.61893)
  line L11 (-27.277537, 78.61893) -> (-27.277537, 80)
  line L12 (-27.277537, 80) -> (-88.000001, 80)
extrude "押し出し41" cut sketch "スケッチ51" along normal blind 73 contours L0 L1 L2 L3 picked at (-74.666668, 19.466667) bodies 1
extrude "押し出し42" add 2 faces at (1, 79.000001, 29.733333) (2, 79.000001, 12.333333) along direction (0, -1, 0) blind 5 on bodies 1 bodies 1
sketch "スケッチ52" plane through (0, 0, 0) normal (-1, 0, 0) x (0, -1, 0)
  line L0 (-82.000001, 28.4) -> (-71.000001, 28.4)
  line L1 (-71.000001, 28.4) -> (-71.000001, 15)
  line L2 (-71.000001, 15) -> (-82.000001, 15)
  line L3 (-82.000001, 15) -> (-82.000001, 28.4)
  line L4 (0, 0) -> (-13.397461, 50)
  line L5 (-13.397461, 50) -> (-21.435937, 80)
  line L6 (-21.435937, 80) -> (-100, 80)
  line L7 (-100, 80) -> (-100, -3)
  line L8 (-100, -3) -> (0, -3)
  line L9 (0, -3) -> (0, 0)
  line L10 (-69.874321, 28.4) -> (-71.000001, 28.4)
  line L11 (-71.000001, 28.4) -> (-71.000001, 15)
  line L12 (-71.000001, 15) -> (-69.874321, 15)
  line L13 (-69.874321, 15) -> (-69.874321, 28.4)
  constraint horizontal L10
  constraint vertical L11
  constraint horizontal L12
  constraint vertical L13
extrude "押し出し43" cut sketch "スケッチ52" against normal blind 85 contours L1 L10 L11 L12 L13 picked at (-70.624774, 23.933333) bodies 1
component "Component" placed x (0, 0, -1) y (0, 1, 0) z (1, 0, 0) at (-99.106277, 0, 65.106278)
